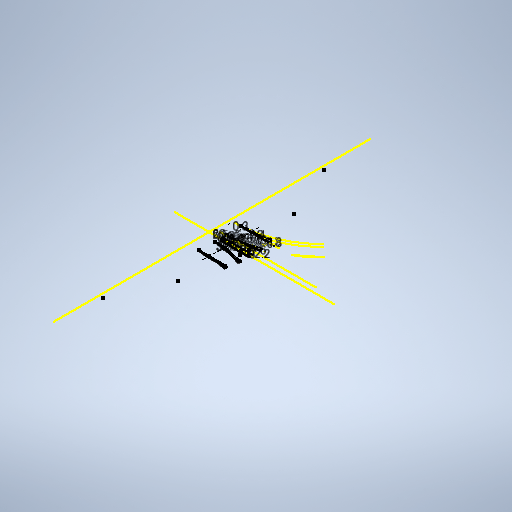
# Autodesk Inventor part: RR_SingleTurnoutLever
Saved by Autodesk Inventor 2025.1 (Build 291241000, 241)
## iProperties
Created: 2025-03-06
Part Number: RR_SingleTurnoutLever
Material: 一般
Document SubType Name: Modeling
Designer: kumagai
Density: 1 g/cm^3
Appearance: 既定
Author: kumagai
Autodesk Inventor part; units mm, degrees
ref_plane "YZ Plane" through (0, 0, 0) normal (1, 0, 0) x (0, 1, 0)
ref_plane "XZ Plane" through (0, 0, 0) normal (0, 1, 0) x (-1, 0, 0)
ref_plane "XY Plane" through (0, 0, 0) normal (0, 0, 1) x (1, 0, 0)
derived "RR_SingleTurnout.ipt"
sketch "MainSketch" plane through (0, 0, 0) normal (0, 1, 0) x (-1, 0, 0)
  line L0 (0, -306.5136) -> (0, 56.9483)
  line L1 (-275.3685, 0) -> (77.2109, 0)
  line L2 (14.6359, -29) -> (-5, -29)
  line L3 (-5, -49.5106) -> (-5, -5.6416)
  line L4 (-5, -48) -> (0, -48)
  line L5 (-5, -10) -> (0, -10)
  line L6 (-5, -38.3) -> (0, -38.3)
  line L7 (-5, -19.7) -> (0, -19.7)
  line L8 (-5, -46) -> (0, -46)
  line L9 (-5, -35.9) -> (0, -35.9)
  line L10 (-5, -22.1) -> (0, -22.1)
  line L11 (-5, -12) -> (0, -12)
  line L12 (-10, -10) -> (-225, -10)
  line L13 (-10, -10) -> (-10, -48)
  line L14 (-225, -48) -> (-225, -10)
  line L15 (-10, -12) -> (-225, -12)
  line L16 (-93.0964, -19.7) -> (-225, -19.7)
  arc A0 (-10, -48) -> (-148.5929, -105.4071) centre (-10, -244) ccw
  arc A1 (-10, -46) -> (-150.0071, -103.9929) centre (-10, -244) ccw
  line L17 (-143.2215, -110.7785) -> (-189.5102, -64.4898)
  line L18 (-210, -35.9) -> (-210, -22.1)
  line L19 (-146.1596, -86.6272) -> (-155.9415, -76.8453)
  arc A2 (-133.8847, -47.8455) -> (-174.0488, -79.9512) centre (-10, -244) ccw
  arc A3 (-139.2229, -48.9168) -> (-175.463, -78.537) centre (-10, -244) ccw
  line L20 (-139.499, -48) -> (-225, -48)
  line L21 (-134.4186, -46) -> (-225, -46)
  arc A4 (-118.9103, -50.6657) -> (-166.907, -87.093) centre (-10, -244) ccw
  arc A5 (-120.0882, -48.5746) -> (-168.6041, -85.3959) centre (-10, -244) ccw
  line L22 (-88.3997, -46) -> (-110.2721, -46)
  arc A6 (-91.8079, -26.9022) -> (-113.1913, -36.2127) centre (-10, -244) ccw
  line L23 (-122.0871, -35.9) -> (-225, -35.9)
  line L24 (-122.0871, -38.3) -> (-225, -38.3)
  arc A7 (-133.8847, -47.8455) -> (-134.4186, -46) centre (-134.4186, -47) ccw
  arc A8 (-139.2229, -48.9168) -> (-139.499, -48) centre (-139.499, -48.5) ccw
  arc A9 (-110.2721, -48.4) -> (-118.9103, -50.6657) centre (-110.2721, -66) ccw
  arc A10 (-110.2721, -46) -> (-120.0882, -48.5746) centre (-110.2721, -66) ccw
  arc A11 (-122.0871, -38.3) -> (-113.1913, -36.2127) centre (-122.0871, -18.3) ccw
  arc A12 (-122.0871, -35.9) -> (-114.2588, -34.0632) centre (-122.0871, -18.3) ccw
  arc A13 (-84.3565, -34.9289) -> (-84.1889, -35.9) centre (-84.1889, -35.4) ccw
  arc A14 (-94.865, -36.3743) -> (-94.4867, -38.3) centre (-94.4867, -37.3) ccw
  arc A15 (-103.9259, -28.5866) -> (-108.3051, -30.5495) centre (-10, -244) ccw
  arc A16 (-92.2005, -21.1444) -> (-91.4727, -25.2405) centre (-89.0652, -22.7) ccw
  arc A17 (-95.2936, -25.6691) -> (-114.2588, -34.0632) centre (-10, -244) ccw
  line L25 (-95.9536, -22.1) -> (-225, -22.1)
  arc A18 (-94.9553, -23.042) -> (-94.7021, -24.4424) centre (-89.0652, -22.7) ccw
  arc A19 (-91.8079, -26.9022) -> (-91.4727, -25.2405) centre (-92.1605, -25.9664) ccw
  arc A20 (-92.2005, -21.1444) -> (-93.0964, -19.7) centre (-93.0964, -20.7) ccw
  arc A21 (-95.2936, -25.6691) -> (-94.7021, -24.4424) centre (-95.6575, -24.7377) ccw
  arc A22 (-94.9553, -23.042) -> (-95.9536, -22.1) centre (-95.9536, -23.1) ccw
  circle A23 centre (-89.0652, -22.7) radius 2.5
  arc A24 (-96.0029, -53.8443) -> (-104.887, -58.1179) centre (-10, -244) ccw
  arc A25 (-90.2587, -49.342) -> (-89.9638, -50.8719) centre (-84.3686, -49) ccw
  arc A26 (-87.5039, -47.4444) -> (-86.7188, -51.5936) centre (-84.3686, -49) ccw
  arc A27 (-90.5252, -52.1112) -> (-157.1489, -96.8511) centre (-10, -244) ccw
  line L26 (-91.257, -48.4) -> (-110.2721, -48.4)
  arc A28 (-87.0159, -53.2618) -> (-155.4519, -98.5481) centre (-10, -244) ccw
  arc A29 (-87.0159, -53.2618) -> (-86.7188, -51.5936) centre (-87.3903, -52.3346) ccw
  arc A30 (-87.5039, -47.4444) -> (-88.3997, -46) centre (-88.3997, -47) ccw
  arc A31 (-90.5252, -52.1112) -> (-89.9638, -50.8719) centre (-90.9121, -51.1891) ccw
  arc A32 (-90.2587, -49.342) -> (-91.257, -48.4) centre (-91.257, -49.4) ccw
  circle A33 centre (-84.3686, -49) radius 2.5
  line L27 (-43.4568, -12) -> (-26.6853, -12)
  arc A34 (-26.6638, -12.5992) -> (-88.0559, -25.5251) centre (-10, -244) ccw
  arc A35 (-89.0652, -19.7) -> (-88.0559, -25.5251) centre (-89.0652, -22.7) ccw
  arc A36 (-26.6638, -12.5992) -> (-26.6853, -12) centre (-26.6853, -12.3) ccw
  arc A37 (-43.4568, -12) -> (-76.6882, -19.2867) centre (-10, -244) ccw
  line L28 (-89.0652, -19.7) -> (-79.5332, -19.7)
  arc A38 (-79.5332, -19.7) -> (-76.6882, -19.2867) centre (-79.5332, -9.7) ccw
  circle A39 centre (-84.3686, -49) radius 3
  line L29 (-84.9577, -46.0584) -> (-27.1511, -34.4821)
  arc A40 (-27.0106, -35.065) -> (-41.7023, -39.8438) centre (26.8424, -225.6007) ccw
  arc A41 (-27.0106, -35.065) -> (-27.1511, -34.4821) centre (-27.0922, -34.7763) ccw
  arc A42 (-74.694, -46.7073) -> (-82.77, -51.5386) centre (26.8424, -225.6007) ccw
  line L30 (-73.2077, -46.153) -> (-41.7023, -39.8438)
  arc A43 (-73.2077, -46.153) -> (-74.694, -46.7073) centre (-72.2259, -51.0557) ccw
  arc A44 (-48.4878, -13.998) -> (-81.6596, -22.083) centre (-10, -244) ccw
  arc A45 (-27.9859, -39.0878) -> (-44.4613, -41.2072) centre (-10, -244) ccw
  line L31 (-33.0916, -19.7) -> (-48.0227, -19.7)
  line L32 (-25.8398, -35.9879) -> (-26.1688, -34.3986)
  line L33 (-26.7598, -34.0104) -> (-46.4779, -38.0924)
  line L34 (-46.9644, -35.7422) -> (-27.2463, -31.6602)
  line L35 (-23.8186, -33.9121) -> (-23.4896, -35.5014)
  line L36 (-10, -38.3) -> (-23, -38.3)
  line L37 (-48.5051, -38.3) -> (-94.4867, -38.3)
  line L38 (-10, -35.9) -> (-23, -35.9)
  line L39 (-48.5051, -35.9) -> (-84.1889, -35.9)
  arc A46 (-25.8398, -35.9879) -> (-23, -38.3) centre (-23, -35.4) ccw
  arc A47 (-23.4896, -35.5014) -> (-23, -35.9) centre (-23, -35.4) ccw
  arc A48 (-23.8186, -33.9121) -> (-27.2463, -31.6602) centre (-26.6584, -34.5) ccw
  arc A49 (-26.1688, -34.3986) -> (-26.7598, -34.0104) centre (-26.6584, -34.5) ccw
  arc A50 (-48.5051, -38.3) -> (-46.4779, -38.0924) centre (-48.5051, -28.3) ccw
  arc A51 (-48.5051, -35.9) -> (-46.9644, -35.7422) centre (-48.5051, -28.3) ccw
  arc A52 (-10, -22.1) -> (-22.0271, -22.4262) centre (-10, -244) ccw
  arc A53 (-46.742, -25.163) -> (-84.3565, -34.9289) centre (-10, -244) ccw
  arc A54 (-10, -19.7) -> (-22.1572, -20.0297) centre (-10, -244) ccw
  arc A55 (-47.1394, -22.7961) -> (-94.865, -36.3743) centre (-10, -244) ccw
  arc A56 (-25.455, -23.997) -> (-45.2368, -22.6611) centre (-50.9626, -254.5905) ccw
  line L40 (-24.9, -22.9254) -> (-24.9, -23.5)
  arc A57 (-25.455, -23.997) -> (-24.9, -23.5) centre (-25.4, -23.5) ccw
  arc A58 (-22.1572, -20.0297) -> (-24.9, -22.9254) centre (-22, -22.9254) ccw
  arc A59 (-45.2368, -22.6611) -> (-47.1394, -22.7961) centre (-45.4836, -32.6581) ccw
  arc A60 (-25.7188, -26.3824) -> (-45.296, -25.0604) centre (-50.9626, -254.5905) ccw
  arc A61 (-22.0271, -22.4262) -> (-22.5, -22.9254) centre (-22, -22.9254) ccw
  line L41 (-22.5, -22.9254) -> (-22.5, -23.5)
  arc A62 (-25.7188, -26.3824) -> (-22.5, -23.5) centre (-25.4, -23.5) ccw
  arc A63 (-45.296, -25.0604) -> (-46.742, -25.163) centre (-45.4836, -32.6581) ccw
  line L42 (-51.7, -52.4873) -> (-51.7, -10)
  line L43 (-44.3, -51.0246) -> (-44.3, -10)
  line L44 (-48, 3.3517) -> (-48, 5.0252)
  line L45 (-59, -53) -> (-37, -53)
  line L46 (-59, -8.2) -> (-37, -8.2)
  line L47 (-37, -8.2) -> (-37, 0.8)
  line L48 (-40, 3.8) -> (-42, 3.8)
  line L49 (-42, 3.8) -> (-40, -7.7)
  line L50 (-40, -7.7) -> (-56, -7.7)
  line L51 (-56, -7.7) -> (-54, 3.8)
  line L52 (-54, 3.8) -> (-56, 3.8)
  line L53 (-59, 0.8) -> (-59, -8.2)
  line L54 (-37, -8.2) -> (-37, -10)
  line L55 (-59, -8.2) -> (-59, -10)
  arc A64 (-37, 0.8) -> (-40, 3.8) centre (-40, 0.8) ccw
  arc A65 (-56, 3.8) -> (-59, 0.8) centre (-56, 0.8) ccw
  line L56 (-44.3, -10) -> (-44.3, -7.7)
  line L57 (-51.7, -10) -> (-51.7, -7.7)
  line L58 (-48, -62.1182) -> (-48, -64.3828)
  line L59 (-37, -53) -> (-37, -62)
  line L60 (-40, -65) -> (-42, -65)
  line L61 (-42, -65) -> (-40, -53.5)
  line L62 (-40, -53.5) -> (-56, -53.5)
  line L63 (-56, -53.5) -> (-54, -65)
  line L64 (-54, -65) -> (-56, -65)
  line L65 (-59, -62) -> (-59, -53)
  arc A66 (-40, -65) -> (-37, -62) centre (-40, -62) ccw
  arc A67 (-59, -62) -> (-56, -65) centre (-56, -62) ccw
  line L66 (-37, -53) -> (-37, -49.8686)
  line L67 (-44.3, -51.0246) -> (-44.3, -53.5)
  line L68 (-51.7, -52.4873) -> (-51.7, -53.5)
  arc A68 (-34.3731, -49.5213) -> (-37, -52.498) centre (-34, -52.498) ccw
  arc A69 (-59, -58.1371) -> (-62.8083, -55.2481) centre (-62, -58.1371) ccw
  arc A70 (-37, -7) -> (-34, -10) centre (-34, -7) ccw
  arc A71 (-62, -10) -> (-59, -7) centre (-62, -7) ccw
  point P0 (0, 0)
  point P1 (-90.868, -19.7)
  point P2 (-94.9346, -22.1)
  point P3 (-90.238, -48.4)
  point P4 (-86.1714, -46)
  point P5 (-162.028, -91.972)
  point P6 (-225, -29)
  point P7 (-10, -29)
  point P8 (-48.5835, -39.998)
  point P9 (-48, 2.002)
  point P10 (-48, -55.998)
  point P11 (-37, 3.8)
  point P12 (-59, 3.8)
  point P13 (-37, -65)
  point P14 (-59, -65)
sketch "LeverSketch" plane through (0, 0, 0) normal (0, 1, 0) x (-1, 0, 0)
  arc A0 (-87.0159, -53.2618) -> (-155.4519, -98.5481) centre (-10, -244) ccw projected
  line L0 (-88.3997, -46) -> (-110.2721, -46) projected
  arc A1 (-10, -46) -> (-150.0071, -103.9929) centre (-10, -244) ccw projected
  arc A2 (-133.8847, -47.8455) -> (-174.0488, -79.9512) centre (-10, -244) ccw projected
  arc A3 (-139.2229, -48.9168) -> (-175.463, -78.537) centre (-10, -244) ccw projected
  line L1 (-10, -12) -> (-225, -12) projected
  circle A4 centre (-84.3686, -49) radius 3
  circle A5 centre (-89.0652, -22.7) radius 3
  arc A6 (-27.3433, -12.6492) -> (-88.0559, -25.5251) centre (-10, -244) ccw
  arc A7 (-27.3433, -12.6492) -> (-27.3657, -12.05) centre (-27.3657, -12.35) ccw
  arc A8 (-43.8017, -12.05) -> (-76.6882, -19.2867) centre (-10, -244) ccw
  line L2 (-43.8017, -12.05) -> (-27.3657, -12.05)
  line L3 (-89.0652, -19.7) -> (-79.5332, -19.7)
  arc A9 (-48.4878, -13.998) -> (-62.7446, -16.8431) centre (-10, -244) ccw
  arc A10 (-79.5332, -19.7) -> (-76.6882, -19.2867) centre (-79.5332, -9.7) ccw
  line L4 (-84.3686, -46) -> (-25.4143, -46)
  line L5 (-60.1893, -48.4) -> (-40.735, -48.4)
  arc A11 (-25.391, -46.5991) -> (-40.735, -48.4) centre (-10, -244) ccw
  arc A12 (-25.391, -46.5991) -> (-25.4143, -46) centre (-25.4143, -46.3) ccw
  line L6 (0, -354.3086) -> (0, 343.7181) projected
  line L7 (-275.3685, 0) -> (77.2109, 0) projected
  circle A13 centre (-89.0652, 22.7) radius 3
  arc A14 (-88.0559, 25.5251) -> (-27.3433, 12.6492) centre (-10, 244) ccw
  arc A15 (-27.3657, 12.05) -> (-27.3433, 12.6492) centre (-27.3657, 12.35) ccw
  arc A16 (-76.6882, 19.2867) -> (-43.8017, 12.05) centre (-10, 244) ccw
  line L8 (-43.8017, 12.05) -> (-27.3657, 12.05)
  line L9 (-89.0652, 19.7) -> (-79.5332, 19.7)
  arc A17 (-76.6882, 19.2867) -> (-79.5332, 19.7) centre (-79.5332, 9.7) ccw
  circle A18 centre (-84.3686, 49) radius 3
  line L10 (-84.3686, 46) -> (-25.4143, 46)
  line L11 (-60.1893, 48.4) -> (-40.735, 48.4)
  arc A19 (-83.4947, 51.8699) -> (-60.1893, 48.4) centre (-60.1893, 128.4) ccw
  arc A20 (-40.735, 48.4) -> (-25.391, 46.5991) centre (-10, 244) ccw
  arc A21 (-25.4143, 46) -> (-25.391, 46.5991) centre (-25.4143, 46.3) ccw
  circle A22 centre (-89.0652, -22.7) radius 1.1
  circle A23 centre (-84.3686, -49) radius 1.1
  circle A24 centre (-89.0652, 22.7) radius 1.1
  circle A25 centre (-84.3686, 49) radius 1.1
  circle A26 centre (-84.3686, -49) radius 2.4
  circle A27 centre (-89.0652, -22.7) radius 2.4
  circle A28 centre (-84.3686, -49) radius 1.65
  circle A29 centre (-89.0652, -22.7) radius 1.65
  circle A30 centre (-48.4878, -13.998) radius 1.6
  circle A31 centre (-47.5125, -47.2) radius 1.6
  circle A32 centre (-48.4878, -13.998) radius 1.8
  circle A33 centre (-47.5125, -47.2) radius 1.8
  circle A34 centre (-48.4878, 13.998) radius 1.65
  circle A35 centre (-48.4878, 13.998) radius 1.85
  circle A36 centre (-47.5125, 47.2) radius 1.65
  circle A37 centre (-47.5125, 47.2) radius 1.85
  line L12 (-60, -5.0418) -> (-60, -4.3264)
  line L13 (-30.5, -3.5) -> (-89.5, -3.5)
  line L14 (-92, -1) -> (-92, 1)
  line L15 (-89.5, 3.5) -> (-30.5, 3.5)
  line L16 (-28, 1) -> (-28, -1)
  arc A38 (-48.4, -1) -> (-45.6, -1) centre (-47, -1) ccw
  arc A39 (-45.6, 1) -> (-48.4, 1) centre (-47, 1) ccw
  line L17 (-45.6, -1) -> (-45.6, 1)
  line L18 (-48.4, -1) -> (-48.4, 1)
  arc A40 (-74.4, -1) -> (-71.6, -1) centre (-73, -1) ccw
  arc A41 (-71.6, 1) -> (-74.4, 1) centre (-73, 1) ccw
  line L19 (-74.4, -1) -> (-74.4, 1)
  line L20 (-71.6, -1) -> (-71.6, 1)
  circle A42 centre (-31, 0) radius 1.6
  circle A43 centre (-89, 0) radius 1.6
  arc A44 (-30.5, -3.5) -> (-28, -1) centre (-30.5, -1) ccw
  arc A45 (-28, 1) -> (-30.5, 3.5) centre (-30.5, 1) ccw
  arc A46 (-89.5, 3.5) -> (-92, 1) centre (-89.5, 1) ccw
  arc A47 (-92, -1) -> (-89.5, -3.5) centre (-89.5, -1) ccw
  arc A48 (-60.1893, -48.4) -> (-83.4947, -51.8699) centre (-60.1893, -128.4) ccw
  point P0 (0, 0)
  point P1 (-78.0652, -19.7)
  point P2 (-25.391, -46.5991)
  point P3 (-46.4542, -46)
  point P4 (-48.5708, -46)
  point P5 (-48.5708, -48.4)
  point P6 (-46.4542, -48.4)
  point P7 (-47.639, -12.6417)
  point P8 (-49.732, -12.9919)
  point P9 (-49.3305, -15.3581)
  point P10 (-47.2483, -15.0097)
  point P11 (-48.8542, -46)
  point P12 (-48.8542, -48.4)
  point P13 (-46.1709, -48.4)
  point P14 (-46.1709, -46)
  point P15 (-50.0119, -13.0402)
  point P16 (-49.609, -15.4062)
  point P17 (-46.9693, -14.9645)
  point P18 (-47.3586, -12.5963)
  point P19 (-46.3801, 48.4)
  point P20 (-48.645, 48.4)
  point P21 (-48.645, 46)
  point P22 (-46.3801, 46)
  point P23 (-47.1753, 14.9978)
  point P24 (-49.4034, 15.3707)
  point P25 (-49.8052, 13.0045)
  point P26 (-47.5656, 12.6298)
  point P27 (-46.1045, 48.4)
  point P28 (-48.9206, 48.4)
  point P29 (-48.9206, 46)
  point P30 (-46.1045, 46)
  point P31 (-46.904, 14.9539)
  point P32 (-49.6742, 15.4175)
  point P33 (-50.0774, 13.0516)
  point P34 (-47.2929, 12.5857)
  point P35 (-47, 2.4)
  point P36 (-47, -2.4)
  dimension "d1" = 6
  dimension "d2" = 6
  dimension "d3" = 0.3
  dimension "d4" = 0.05
  dimension "d5" = 1.2
  dimension "d24" = 2.4
  dimension "d25" = 10
  dimension "d31" = 2.4
  dimension "d61" = 0.3
  dimension "d64" = 1.2
  dimension "d69" = 41.5
  dimension "d70" = 36.9
  dimension "d71" = 2.2
  dimension "d72" = 4.8
  dimension "d81" = 3.3
  dimension "d84" = 3.2
  dimension "d85" = 3.6
  dimension "d90" = 3.3
  dimension "d91" = 3.7
  dimension "d102" = 60
  dimension "d118" = 2.8
  dimension "d119" = 26
  dimension "d120" = 4.8
  dimension "d121" = 7
  dimension "d122" = 1.1
  dimension "d123" = 16
  dimension "d124" = 3.2
  dimension "d125" = 16
  dimension "d127" = 3
  dimension "d128" = 3
  dimension "d129" = 2.5
  dimension "d130" = 80
  constraints: 58 point on circle, 45 centre point, 35 end point, 29 symmetric about line, 23 coincident, 22 tangent, 14 equal radius, 4 vertical, 3 parallel, 3 point on line, 1 collinear, 14 other
  measures "d1" diameter of A4
  measures "d2" diameter of A5
  measures "d3" radius of A7
  measures "d4" distance between parallel lines of L1 L2
  measures "d5" radial gap between concentric circles of A8 A9
  measures "d24" radial gap between concentric circles of A8 A6
  measures "d25" radius of A10
  measures "d31" distance between parallel lines of L4 L5
  measures "d61" radius of A12
  measures "d64" distance from line of L4 point (-47.513, -47.2)
  measures "d69" distance of point (-48.488, -13.998) point (-89.065, -22.7)
  measures "d70" distance of point (-84.369, -49) point (-47.513, -47.2)
  measures "d71" diameter of A22
  measures "d72" diameter of A26
  measures "d81" diameter of A28
  measures "d84" diameter of A30
  measures "d85" diameter of A32
  measures "d90" diameter of A34
  measures "d91" diameter of A35
  measures "d102" distance between parallel lines of L6 L12
  measures "d118" distance between parallel lines of L18 L17
  measures "d119" distance of A40.centre A38.centre
  measures "d120" distance of point (-47, 2.4) point (-47, -2.4)
  measures "d121" distance between parallel lines of L15 L13
  measures "d122" distance from line of L13 point (-47, -2.4)
  measures "d123" horizontal distance of A42.centre A38.centre
  measures "d124" diameter of A42
  measures "d125" horizontal distance of A43.centre A40.centre
  measures "d127" distance from line of L16 A42.centre
  measures "d128" distance from line of L14 A43.centre
  measures "d129" radius of A44
  measures "d130" radius of A48
extrude "LeverBody" add sketch "LeverSketch" against normal blind 2.8 contours A1 L5 A33 L4 A12 | L5 A31 L4 A33 | L5 A31 L4 | A33 L4 A31 L5 | L5 A48 A4 L4 A33 | A4 | A5 | A5 L3 A10 A8 A32 A6 | A32 A9 A30 A6 | A30 A8 A6 | A32 A8 A30 A9 | A32 A8 L2 A7 A6 | A6 A30 A8 A32 | A13 | A13 A14 A35 A16 A17 L9 | A14 A34 A16 A35 | A14 A34 A16 | A35 A16 A34 A14 | A14 A15 L8 A16 A35 | A18 | A18 A19 L11 A37 L10 | A37 L11 A36 L10 | A36 L11 L10 | A37 L11 A20 A21 L10 | L10 A36 L11 A37 | A26 | A27 | A28 | A29
extrude "Boss" add sketch "LeverSketch" along normal blind 2.8 contours A26 | A27 | A28 | A29
chamfer "ScrewDish" distance 1.2 angle 45 2 edges at (90.1652, -2.8, 22.7) (85.4686, -2.8, 49)
extrude "InsertHole" cut sketch "LeverSketch" along normal blind 3.4 from surface at -2.8 contours A28 | A29
chamfer "InsertChamfer" distance 0.4 angle 45 2 edges at (86.0186, -2.8, -49) (90.7152, -2.8, -22.7)
extrude "Pin" add sketch "LeverSketch" along normal blind 2.8 contours L5 A31 L4 | A30 A8 A6
extrude "Hat" add sketch "LeverSketch" along normal blind 0.4 from surface at 2.8 contours L5 A31 L4 A33 | L5 A31 L4 | A33 L4 A31 L5 | A32 A9 A30 A6 | A30 A8 A6 | A32 A8 A30 A9 | A6 A30 A8 A32
extrude "SlotP" cut sketch "LeverSketch" against normal blind 0.4 contours A14 A34 A16 | A36 L11 L10
extrude "SlotH" cut sketch "LeverSketch" against normal blind 0.4 from surface at -0.4 contours A14 A34 A16 A35 | A14 A34 A16 | A35 A16 A34 A14 | A37 L11 A36 L10 | A36 L11 L10 | L10 A36 L11 A37
extrude "SlidePlate" add sketch "LeverSketch" along normal blind 2 from surface at -2.8 contours L14 A46 L15 A45 L16 L7 A42 L17 A39 L18 L20 A41 L19 A43 | L7 A43 L19 A40 L20 L18 A38 L17 A42 L16 A44 L13 A47 L14
equation "\"d5\" = 0.5 * InnerWall"
equation "\"d24\" = InnerWall"
equation "\"d31\" = InnerWall"
equation "\"d64\" = 0.5 * InnerWall"
equation "\"InnerWall\" = 2.4"
